Autodesk Fusion 360 part; units mm, degrees
(part 6 of 6)
  line L2217 (-53.3431, 39) -> (-51, 36.6569)
  line L2218 (-51, 36.6569) -> (-51, 33.3431)
  line L2219 (-51, 33.3431) -> (-53.3431, 31)
  line L2220 (-53.3431, 31) -> (-56.6569, 31)
  line L2221 (-56.6569, 31) -> (-59, 33.3431)
  line L2222 (-49, 33.3431) -> (-49, 36.6569)
  line L2223 (-49, 36.6569) -> (-46.6569, 39)
  line L2224 (-46.6569, 39) -> (-43.3431, 39)
  line L2225 (-43.3431, 39) -> (-41, 36.6569)
  line L2226 (-41, 36.6569) -> (-41, 33.3431)
  line L2227 (-41, 33.3431) -> (-43.3431, 31)
  line L2228 (-43.3431, 31) -> (-46.6569, 31)
  line L2229 (-46.6569, 31) -> (-49, 33.3431)
  line L2230 (-39, 33.3431) -> (-39, 36.6569)
  line L2231 (-39, 36.6569) -> (-36.6569, 39)
  line L2232 (-36.6569, 39) -> (-33.3431, 39)
  line L2233 (-33.3431, 39) -> (-31, 36.6569)
  line L2234 (-31, 36.6569) -> (-31, 33.3431)
  line L2235 (-31, 33.3431) -> (-33.3431, 31)
  line L2236 (-33.3431, 31) -> (-36.6569, 31)
  line L2237 (-36.6569, 31) -> (-39, 33.3431)
  line L2238 (-29, 33.3431) -> (-29, 36.6569)
  line L2239 (-29, 36.6569) -> (-26.6569, 39)
  line L2240 (-26.6569, 39) -> (-23.3431, 39)
  line L2241 (-23.3431, 39) -> (-21, 36.6569)
  line L2242 (-21, 36.6569) -> (-21, 33.3431)
  line L2243 (-21, 33.3431) -> (-23.3431, 31)
  line L2244 (-23.3431, 31) -> (-26.6569, 31)
  line L2245 (-26.6569, 31) -> (-29, 33.3431)
  line L2246 (-19, 33.3431) -> (-19, 36.6569)
  line L2247 (-19, 36.6569) -> (-16.6569, 39)
  line L2248 (-16.6569, 39) -> (-13.3431, 39)
  line L2249 (-13.3431, 39) -> (-11, 36.6569)
  line L2250 (-11, 36.6569) -> (-11, 33.3431)
  line L2251 (-11, 33.3431) -> (-13.3431, 31)
  line L2252 (-13.3431, 31) -> (-16.6569, 31)
  line L2253 (-16.6569, 31) -> (-19, 33.3431)
  line L2254 (-9, 33.3431) -> (-9, 36.6569)
  line L2255 (-9, 36.6569) -> (-6.6569, 39)
  line L2256 (-6.6569, 39) -> (-3.3431, 39)
  line L2257 (-3.3431, 39) -> (-1, 36.6569)
  line L2258 (-1, 36.6569) -> (-1, 33.3431)
  line L2259 (-1, 33.3431) -> (-3.3431, 31)
  line L2260 (-3.3431, 31) -> (-6.6569, 31)
  line L2261 (-6.6569, 31) -> (-9, 33.3431)
  line L2262 (1, 33.3431) -> (1, 36.6569)
  line L2263 (1, 36.6569) -> (3.3431, 39)
  line L2264 (3.3431, 39) -> (6.6569, 39)
  line L2265 (6.6569, 39) -> (9, 36.6569)
  line L2266 (9, 36.6569) -> (9, 33.3431)
  line L2267 (9, 33.3431) -> (6.6569, 31)
  line L2268 (6.6569, 31) -> (3.3431, 31)
  line L2269 (3.3431, 31) -> (1, 33.3431)
  line L2270 (11, 33.3431) -> (11, 36.6569)
  line L2271 (11, 36.6569) -> (13.3431, 39)
  line L2272 (13.3431, 39) -> (16.6569, 39)
  line L2273 (16.6569, 39) -> (19, 36.6569)
  line L2274 (19, 36.6569) -> (19, 33.3431)
  line L2275 (19, 33.3431) -> (16.6569, 31)
  line L2276 (16.6569, 31) -> (13.3431, 31)
  line L2277 (13.3431, 31) -> (11, 33.3431)
  line L2278 (21, 33.3431) -> (21, 36.6569)
  line L2279 (21, 36.6569) -> (23.3431, 39)
  line L2280 (23.3431, 39) -> (26.6569, 39)
  line L2281 (26.6569, 39) -> (29, 36.6569)
  line L2282 (29, 36.6569) -> (29, 33.3431)
  line L2283 (29, 33.3431) -> (26.6569, 31)
  line L2284 (26.6569, 31) -> (23.3431, 31)
  line L2285 (23.3431, 31) -> (21, 33.3431)
  line L2286 (31, 33.3431) -> (31, 36.6569)
  line L2287 (31, 36.6569) -> (33.3431, 39)
  line L2288 (33.3431, 39) -> (36.6569, 39)
  line L2289 (36.6569, 39) -> (39, 36.6569)
  line L2290 (39, 36.6569) -> (39, 33.3431)
  line L2291 (39, 33.3431) -> (36.6569, 31)
  line L2292 (36.6569, 31) -> (33.3431, 31)
  line L2293 (33.3431, 31) -> (31, 33.3431)
  line L2294 (41, 33.3431) -> (41, 36.6569)
  line L2295 (41, 36.6569) -> (43.3431, 39)
  line L2296 (43.3431, 39) -> (46.6569, 39)
  line L2297 (46.6569, 39) -> (49, 36.6569)
  line L2298 (49, 36.6569) -> (49, 33.3431)
  line L2299 (49, 33.3431) -> (46.6569, 31)
  line L2300 (46.6569, 31) -> (43.3431, 31)
  line L2301 (43.3431, 31) -> (41, 33.3431)
  line L2302 (51, 33.3431) -> (51, 36.6569)
  line L2303 (51, 36.6569) -> (53.3431, 39)
  line L2304 (53.3431, 39) -> (56.6569, 39)
  line L2305 (56.6569, 39) -> (59, 36.6569)
  line L2306 (59, 36.6569) -> (59, 33.3431)
  line L2307 (59, 33.3431) -> (56.6569, 31)
  line L2308 (56.6569, 31) -> (53.3431, 31)
  line L2309 (53.3431, 31) -> (51, 33.3431)
  line L2310 (61, 33.3431) -> (61, 36.6569)
  line L2311 (61, 36.6569) -> (63.3431, 39)
  line L2312 (63.3431, 39) -> (66.6569, 39)
  line L2313 (66.6569, 39) -> (69, 36.6569)
  line L2314 (69, 36.6569) -> (69, 33.3431)
  line L2315 (69, 33.3431) -> (66.6569, 31)
  line L2316 (66.6569, 31) -> (63.3431, 31)
  line L2317 (63.3431, 31) -> (61, 33.3431)
  line L2318 (-69, 43.3431) -> (-69, 46.6569)
  line L2319 (-69, 46.6569) -> (-66.6569, 49)
  line L2320 (-66.6569, 49) -> (-63.3431, 49)
  line L2321 (-63.3431, 49) -> (-61, 46.6569)
  line L2322 (-61, 46.6569) -> (-61, 43.3431)
  line L2323 (-61, 43.3431) -> (-63.3431, 41)
  line L2324 (-63.3431, 41) -> (-66.6569, 41)
  line L2325 (-66.6569, 41) -> (-69, 43.3431)
  line L2326 (-59, 43.3431) -> (-59, 46.6569)
  line L2327 (-59, 46.6569) -> (-56.6569, 49)
  line L2328 (-56.6569, 49) -> (-53.3431, 49)
  line L2329 (-53.3431, 49) -> (-51, 46.6569)
  line L2330 (-51, 46.6569) -> (-51, 43.3431)
  line L2331 (-51, 43.3431) -> (-53.3431, 41)
  line L2332 (-53.3431, 41) -> (-56.6569, 41)
  line L2333 (-56.6569, 41) -> (-59, 43.3431)
  line L2334 (-49, 43.3431) -> (-49, 46.6569)
  line L2335 (-49, 46.6569) -> (-46.6569, 49)
  line L2336 (-46.6569, 49) -> (-43.3431, 49)
  line L2337 (-43.3431, 49) -> (-41, 46.6569)
  line L2338 (-41, 46.6569) -> (-41, 43.3431)
  line L2339 (-41, 43.3431) -> (-43.3431, 41)
  line L2340 (-43.3431, 41) -> (-46.6569, 41)
  line L2341 (-46.6569, 41) -> (-49, 43.3431)
  line L2342 (-39, 43.3431) -> (-39, 46.6569)
  line L2343 (-39, 46.6569) -> (-36.6569, 49)
  line L2344 (-36.6569, 49) -> (-33.3431, 49)
  line L2345 (-33.3431, 49) -> (-31, 46.6569)
  line L2346 (-31, 46.6569) -> (-31, 43.3431)
  line L2347 (-31, 43.3431) -> (-33.3431, 41)
  line L2348 (-33.3431, 41) -> (-36.6569, 41)
  line L2349 (-36.6569, 41) -> (-39, 43.3431)
  line L2350 (-29, 43.3431) -> (-29, 46.6569)
  line L2351 (-29, 46.6569) -> (-26.6569, 49)
  line L2352 (-26.6569, 49) -> (-23.3431, 49)
  line L2353 (-23.3431, 49) -> (-21, 46.6569)
  line L2354 (-21, 46.6569) -> (-21, 43.3431)
  line L2355 (-21, 43.3431) -> (-23.3431, 41)
  line L2356 (-23.3431, 41) -> (-26.6569, 41)
  line L2357 (-26.6569, 41) -> (-29, 43.3431)
  line L2358 (-19, 43.3431) -> (-19, 46.6569)
  line L2359 (-19, 46.6569) -> (-16.6569, 49)
  line L2360 (-16.6569, 49) -> (-13.3431, 49)
  line L2361 (-13.3431, 49) -> (-11, 46.6569)
  line L2362 (-11, 46.6569) -> (-11, 43.3431)
  line L2363 (-11, 43.3431) -> (-13.3431, 41)
  line L2364 (-13.3431, 41) -> (-16.6569, 41)
  line L2365 (-16.6569, 41) -> (-19, 43.3431)
  line L2366 (-9, 43.3431) -> (-9, 46.6569)
  line L2367 (-9, 46.6569) -> (-6.6569, 49)
  line L2368 (-6.6569, 49) -> (-3.3431, 49)
  line L2369 (-3.3431, 49) -> (-1, 46.6569)
  line L2370 (-1, 46.6569) -> (-1, 43.3431)
  line L2371 (-1, 43.3431) -> (-3.3431, 41)
  line L2372 (-3.3431, 41) -> (-6.6569, 41)
  line L2373 (-6.6569, 41) -> (-9, 43.3431)
  line L2374 (1, 43.3431) -> (1, 46.6569)
  line L2375 (1, 46.6569) -> (3.3431, 49)
  line L2376 (3.3431, 49) -> (6.6569, 49)
  line L2377 (6.6569, 49) -> (9, 46.6569)
  line L2378 (9, 46.6569) -> (9, 43.3431)
  line L2379 (9, 43.3431) -> (6.6569, 41)
  line L2380 (6.6569, 41) -> (3.3431, 41)
  line L2381 (3.3431, 41) -> (1, 43.3431)
  line L2382 (11, 43.3431) -> (11, 46.6569)
  line L2383 (11, 46.6569) -> (13.3431, 49)
  line L2384 (13.3431, 49) -> (16.6569, 49)
  line L2385 (16.6569, 49) -> (19, 46.6569)
  line L2386 (19, 46.6569) -> (19, 43.3431)
  line L2387 (19, 43.3431) -> (16.6569, 41)
  line L2388 (16.6569, 41) -> (13.3431, 41)
  line L2389 (13.3431, 41) -> (11, 43.3431)
  line L2390 (21, 43.3431) -> (21, 46.6569)
  line L2391 (21, 46.6569) -> (23.3431, 49)
  line L2392 (23.3431, 49) -> (26.6569, 49)
  line L2393 (26.6569, 49) -> (29, 46.6569)
  line L2394 (29, 46.6569) -> (29, 43.3431)
  line L2395 (29, 43.3431) -> (26.6569, 41)
  line L2396 (26.6569, 41) -> (23.3431, 41)
  line L2397 (23.3431, 41) -> (21, 43.3431)
  line L2398 (-70, -47.0711) -> (-67.0711, -50)
  line L2399 (-67.0711, -50) -> (-70, -52.9289)
  line L2400 (-70, -52.9289) -> (-70, -47.0711)
  line L2401 (-67.0711, -70) -> (-70, -70)
  line L2402 (-70, -70) -> (-70, -67.0711)
  line L2403 (-70, -67.0711) -> (-67.0711, -70)
  line L2404 (-63.3431, -61) -> (-61, -63.3431)
  line L2405 (-61, -63.3431) -> (-61, -66.6569)
  line L2406 (-61, -66.6569) -> (-63.3431, -69)
  line L2407 (-63.3431, -69) -> (-66.6569, -69)
  line L2408 (-66.6569, -69) -> (-69, -66.6569)
  line L2409 (-69, -66.6569) -> (-69, -63.3431)
  line L2410 (-69, -63.3431) -> (-66.6569, -61)
  line L2411 (-66.6569, -61) -> (-63.3431, -61)
  line L2412 (-75, 75) -> (-75, -75)
  line L2413 (-75, -75) -> (75, -75)
  line L2414 (75, -75) -> (75, 75)
  line L2415 (75, 75) -> (-75, 75)
  line L2416 (-75, 75) -> (-70, 75)
  line L2417 (-70, 75) -> (-70, 70)
  line L2418 (-70, 70) -> (-75, 70)
  line L2419 (-75, 70) -> (-75, 75)
  line L2420 (70, 70) -> (75, 70)
  line L2421 (75, 70) -> (75, 75)
  line L2422 (75, 75) -> (70, 75)
  line L2423 (70, 75) -> (70, 70)
  line L2424 (70, -70) -> (75, -70)
  line L2425 (75, -70) -> (75, -75)
  line L2426 (75, -75) -> (70, -75)
  line L2427 (70, -75) -> (70, -70)
  line L2428 (-75, -75) -> (-70, -75)
  line L2429 (-70, -75) -> (-70, -70)
  line L2430 (-70, -70) -> (-75, -70)
  line L2431 (-75, -70) -> (-75, -75)
  constraint horizontal L2416
  constraint vertical L2417
  constraint horizontal L2418
  constraint vertical L2419
  constraint coincident L131.end L132.start
  constraint coincident L2412.start L2415.end
  constraint horizontal L2420
  constraint vertical L2421
  constraint horizontal L2422
  constraint vertical L2423
  constraint coincident L2414.end L2415.start
  constraint coincident L89.end L90.start
  constraint horizontal L2424
  constraint vertical L2425
  constraint horizontal L2426
  constraint vertical L2427
  constraint coincident L2413.end L2414.start
  constraint coincident L47.end L48.start
  constraint horizontal L2428
  constraint vertical L2429
  constraint horizontal L2430
  constraint vertical L2431
  constraint coincident L2401.end L2402.start
  constraint coincident L2412.end L2413.start
extrude "Extrude3" add sketch "Sketch2" along normal blind 15 contours L2413 L2414 L2424 L2425 L2426 L2427 | L2414 L2415 L2420 L2421 L2422 L2423 | L2412 L2413 L2428 L2429 L2430 L2431 | L2412 L2415 L2416 L2417 L2418 L2419
extrude "Extrude4" add sketch "Sketch1" along normal blind 1 and the other way blind 15 contours L1316 L1329 L1528 L1530 | L536 L549 L748 L750 | L1376 L1389 L1588 L1590 | L2216 L2229 L2428 L2430 | L1436 L1449 L1648 L1650
